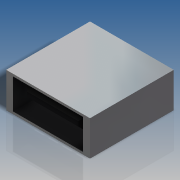
# Autodesk Inventor part: 11032-Black
Saved by Autodesk Inventor 2016 SP2 (Build 200236200, 236)
## iProperties
Created: 2015-08-21
Part Number: 11032-Black
Material: ABS Plastic
Document SubType Name: Modeling
Designer: D. Kohfeld
Density: 1.06 g/cm^3
Appearance: Black
Mass: 0.625925 g
Surface Area: 15.0946 cm^2
Volume: 0.590495 cm^3
Author: D. Kohfeld
Autodesk Inventor part; units mm, degrees
ref_plane "YZ Plane" through (0, 0, 0) normal (1, 0, 0) x (0, 1, 0)
ref_plane "XZ Plane" through (0, 0, 0) normal (0, 1, 0) x (-1, 0, 0)
ref_plane "XY Plane" through (0, 0, 0) normal (0, 0, 1) x (1, 0, 0)
sketch "Sketch2" plane through (0, 0, 0) normal (0, 0, 1) x (1, 0, 0)
  line L0 (-6, 2.6) -> (6, 2.6)
  line L1 (6, 2.6) -> (6, -2.6)
  line L2 (6, -2.6) -> (-6, -2.6)
  line L3 (-6, -2.6) -> (-6, 2.6)
  line L4 (-7.2, 3) -> (7.2, 3)
  line L5 (7.2, 3) -> (7.2, -3)
  line L6 (7.2, -3) -> (-7.2, -3)
  line L7 (-7.2, -3) -> (-7.2, 3)
  point P0 (0, 0)
  point P1 (0, 2.6)
  point P2 (-6, 0)
  point P3 (-7.2, 0)
  point P4 (0, 3)
  dimension "d0" = 5.2
  dimension "d1" = 12
  dimension "d23" = 6
  dimension "d24" = 14.4
  constraints: 16 end point, 4 midpoint, 4 parallel, 2 horizontal, 2 horizontal alignment, 2 perpendicular, 2 vertical alignment
  measures "d0" distance of L2.end L0.start
  measures "d1" distance of L0.start L0.end
  measures "d23" distance of L6.end L4.start
  measures "d24" distance of L4.start L4.end
extrude "Extrusion1" add sketch "Sketch2" along normal mid plane 14.4 contours L0 L1 L2 L3 | L4 L5 L6 L7
sketch "Sketch3" plane through (0, 0, 7.2) normal (0, 0, 1) x (1, 0, 0)
  line L0 (-4.8, 1.158) -> (4.8, 1.158)
  line L1 (4.8, 1.158) -> (4.8, -0.442)
  line L2 (4.8, -0.442) -> (-4.8, -0.442)
  line L3 (-4.8, -0.442) -> (-4.8, 1.158)
  line L4 (-6, 2.6) -> (6, 2.6) projected
  line L5 (-6, -2.6) -> (-6, 2.6) projected
  line L6 (6, -2.6) -> (-6, -2.6) projected
  line L7 (6, 2.6) -> (6, -2.6) projected
  point P0 (0, 0)
  point P1 (0, -0.442)
  dimension "d4" = 1.6
  dimension "d5" = 9.6
  dimension "d25" = 0.442
  constraints: 8 end point, 2 parallel, 1 horizontal, 1 midpoint, 1 perpendicular, 1 vertical alignment
  measures "d4" distance between parallel lines of L2 L0
  measures "d5" distance of L0.start L0.end
  measures "d25" distance from line of point (0, 0) L2
extrude "Extrusion2" cut sketch "Sketch3" against normal blind 13.6
extrude "Extrusion3" cut sketch "Sketch3" against normal blind 0.8 contours L0 L1 L2 L3
chamfer "Chamfer1" distance 0.4 angle 45 4 edges at (-4.8, 0.358, 6.4) (0, 1.158, 6.4) (0, -0.442, 6.4) (4.8, 0.358, 6.4)
sketch "Sketch4" plane through (-4.8, -0.442, -6.4) normal (0, -1, 0) x (1, 0, 0)
  line L0 (0, 0) -> (9.6, 0) projected
  line L1 (0.4, 11.58) -> (2, 11.58)
  line L2 (2, 11.58) -> (2, 0)
  line L3 (2, 0) -> (0.4, 0)
  line L4 (0.4, 0) -> (0.4, 11.58)
  line L5 (2.8, 11.58) -> (4.4, 11.58)
  line L6 (4.4, 11.58) -> (4.4, 0)
  line L7 (4.4, 0) -> (2.8, 0)
  line L8 (2.8, 0) -> (2.8, 11.58)
  line L9 (5.2, 11.58) -> (6.8, 11.58)
  line L10 (6.8, 11.58) -> (6.8, 0)
  line L11 (6.8, 0) -> (5.2, 0)
  line L12 (5.2, 0) -> (5.2, 11.58)
  line L13 (7.6, 11.58) -> (9.2, 11.58)
  line L14 (9.2, 11.58) -> (9.2, 0)
  line L15 (9.2, 0) -> (7.6, 0)
  line L16 (7.6, 0) -> (7.6, 11.58)
  line L17 (2, 11.58) -> (2.8, 11.58) construction
  line L18 (4.4, 11.58) -> (5.2, 11.58) construction
  line L19 (6.8, 11.58) -> (7.6, 11.58) construction
  point P0 (4.8, 6.4)
  point P1 (4.8, 11.58)
  dimension "d18" = 11.58
  dimension "d19" = 1.6
  dimension "d20" = 0.8
  constraints: 38 end point, 8 parallel, 7 horizontal, 5 collinear, 4 perpendicular, 4 point on line, 1 midpoint, 1 vertical alignment
  measures "d18" distance of L3.end L1.start
  measures "d19" distance of L1.start L1.end
  measures "d20" distance between parallel lines of L12 L6
extrude "Extrusion4" add sketch "Sketch4" along normal blind 0.001
equation "\"d4\" = wall"
equation "\"wall\" = 1.6"
body "Solid1"
